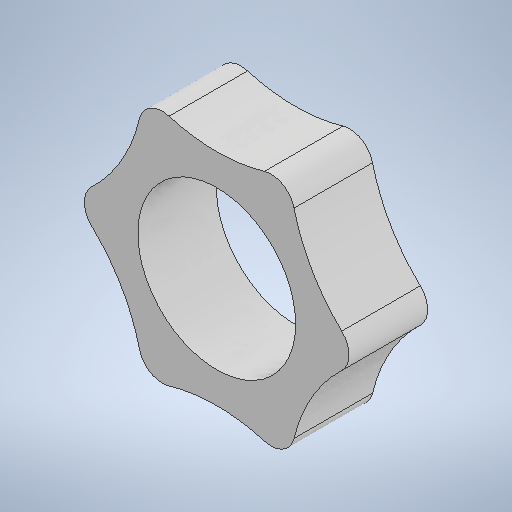
# Autodesk Inventor part: Tool-Lock-Knob
Saved by Autodesk Inventor 2025.3 (Build 293356030, 356C)
## iProperties
Created: 2025-10-10
Part Number: Tool-Lock-Knob
Material: Generic
Document SubType Name: Modeling
Designer: tvoko
Density: 1 g/cm^3
Appearance: Default
Author: tvoko
Autodesk Inventor part; units mm, degrees
ref_plane "YZ Plane" through (0, 0, 0) normal (1, 0, 0) x (0, 1, 0)
ref_plane "XZ Plane" through (0, 0, 0) normal (0, 1, 0) x (-1, 0, 0)
ref_plane "XY Plane" through (0, 0, 0) normal (0, 0, 1) x (1, 0, 0)
sketch "Sketch1" plane through (0, 0, 0) normal (0, 0, 1) x (1, 0, 0)
  circle A0 centre (0, 0) radius 10.05
  line L0 (-8.6603, -15) -> (-17.3205, 0) construction
  line L1 (-17.3205, 0) -> (-8.6603, 15) construction
  line L2 (-8.6603, 15) -> (8.6603, 15) construction
  line L3 (8.6603, 15) -> (17.3205, 0) construction
  line L4 (17.3205, 0) -> (8.6603, -15) construction
  line L5 (8.6603, -15) -> (-8.6603, -15) construction
  arc A1 (6.9282, 15) -> (6.0799, 14.8776) centre (6.9282, 12) ccw
  arc A2 (-6.0799, 14.8776) -> (-9.5263, 13.5) centre (-6.9282, 12) ccw
  arc A3 (-6.0799, 14.8776) -> (6.0799, 14.8776) centre (0, 35.5) ccw
  circle A4 centre (0, 0) radius 14 construction
  arc A5 (-15.9243, 2.1735) -> (-9.8444, 12.7041) centre (-30.7439, 17.75) ccw
  arc A6 (-15.9243, 2.1735) -> (-16.4545, -1.5) centre (-13.8564, 0) ccw
  arc A7 (-9.5263, 13.5) -> (-9.8444, 12.7041) centre (-6.9282, 12) ccw
  arc A8 (-9.8444, -12.7041) -> (-15.9243, -2.1735) centre (-30.7439, -17.75) ccw
  arc A9 (-9.8444, -12.7041) -> (-6.9282, -15) centre (-6.9282, -12) ccw
  arc A10 (-16.4545, -1.5) -> (-15.9243, -2.1735) centre (-13.8564, 0) ccw
  arc A11 (6.0799, -14.8776) -> (-6.0799, -14.8776) centre (0, -35.5) ccw
  arc A12 (6.0799, -14.8776) -> (9.5263, -13.5) centre (6.9282, -12) ccw
  arc A13 (-6.9282, -15) -> (-6.0799, -14.8776) centre (-6.9282, -12) ccw
  arc A14 (15.9243, -2.1735) -> (9.8444, -12.7041) centre (30.7439, -17.75) ccw
  arc A15 (15.9243, -2.1735) -> (16.4545, 1.5) centre (13.8564, 0) ccw
  arc A16 (9.5263, -13.5) -> (9.8444, -12.7041) centre (6.9282, -12) ccw
  arc A17 (9.8444, 12.7041) -> (15.9243, 2.1735) centre (30.7439, 17.75) ccw
  arc A18 (9.8444, 12.7041) -> (6.9282, 15) centre (6.9282, 12) ccw
  arc A19 (16.4545, 1.5) -> (15.9243, 2.1735) centre (13.8564, 0) ccw
  point P0 (-16.4545, -1.5)
  point P1 (-6.9282, -15)
  point P2 (9.5263, -13.5)
  point P3 (16.4545, 1.5)
  dimension "d0" = 20.1
  dimension "d1" = 30
  dimension "d4" = 3
  dimension "d5" = 28
  dimension "d8" = 360
  constraints: 48 point on circle, 20 centre point, 12 end point, 7 tangent, 3 coincident, 2 point on line, 1 equal radius, 1 horizontal, 74 other
  measures "d0" diameter of A0
  measures "d1" distance between parallel lines of L5 L2
  measures "d4" radius of A2
  measures "d5" diameter of A4
extrude "Extrusion1" add sketch "Sketch1" along normal blind 10
body "Solid1"
